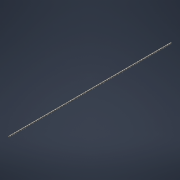
# Autodesk Inventor part: LinearRail
Saved by Autodesk Inventor 2021 (Build 250183000, 183)
## iProperties
Created: 2021-01-30
Part Number: LinearRail
Material: Generic
Document SubType Name: Modeling
Designer: argon
Density: 1 g/cm^3
Appearance: Default
Author: argon
Autodesk Inventor part; units mm, degrees
ref_plane "YZ Plane" through (0, 0, 0) normal (1, 0, 0) x (0, 1, 0)
ref_plane "XZ Plane" through (0, 0, 0) normal (0, 1, 0) x (-1, 0, 0)
ref_plane "XY Plane" through (0, 0, 0) normal (0, 0, 1) x (1, 0, 0)
sketch "Sketch1" plane through (0, 0, 0) normal (0, 0, 1) x (1, 0, 0)
  line L0 (-3, 3) -> (3, 3)
  line L1 (3, 3) -> (3, -3)
  line L2 (3, -3) -> (-3, -3)
  line L3 (-3, -3) -> (-3, 3)
  line L4 (-3, 3) -> (3, -3) construction
  line L5 (3, 3) -> (-3, -3) construction
  line L6 (0, 1) -> (3, 1)
  line L7 (3, 1) -> (3, -1)
  line L8 (3, -1) -> (0, -1)
  line L9 (0, -1) -> (0, 1)
  line L10 (0, 1) -> (3, -1) construction
  line L11 (3, 1) -> (0, -1) construction
  line L12 (0, 1) -> (0, 2)
  line L13 (0, 2) -> (1.5, 0)
  line L14 (0, -1) -> (0, -2)
  line L15 (0, -2) -> (1.5, 0)
  point P0 (0, 0)
  point P1 (0.75, -1)
  point P2 (0.75, 1)
  dimension "d0" = 6
  dimension "d1" = 2
  dimension "d2" = 3
  dimension "d3" = 1
  constraints: 32 end point, 4 midpoint, 4 parallel, 2 equal length, 2 horizontal, 2 perpendicular, 2 vertical, 1 horizontal alignment, 1 point on line
  measures "d0" distance of L0.start L0.end
  measures "d1" distance of L8.end L6.start
  measures "d2" distance of L7.end L8.end
  measures "d3" distance of L8.end L14.end
extrude "Extrusion1" add sketch "Sketch1" along normal blind 1000 contours L0 L1 L6 L13 L12 L9 L14 L15 L8 L2 L3
chamfer "Chamfer1" distance 1 angle 45 2 edges at (3, 1, 500) (3, -1, 500)
body "Solid1"
